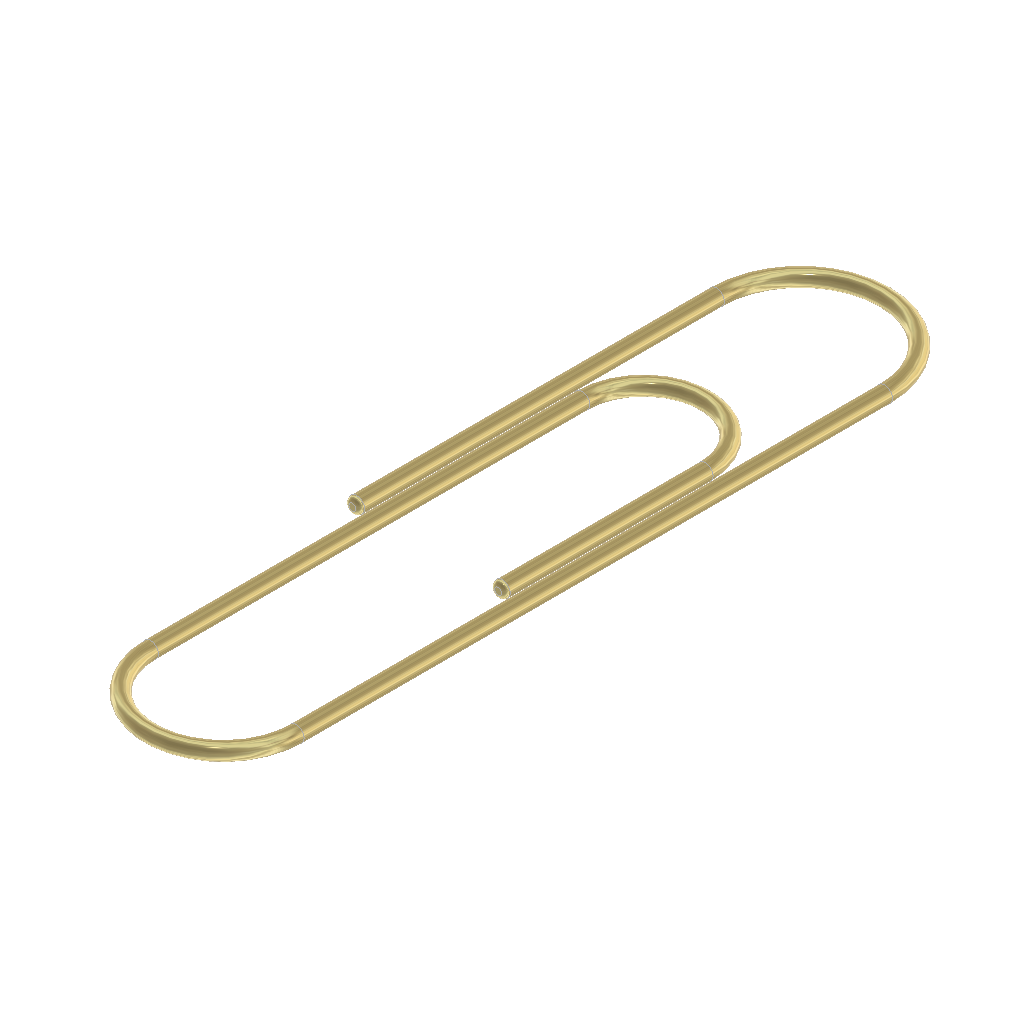
Paper Clip (Autodesk Fusion 360 design; units mm, degrees)
part number: 2026-09-26-18-15-15-186
Autodesk Fusion 360 part; units mm, degrees
sketch "path" plane through (0, 0, 0) normal (0, 0, 1) x (1, 0, 0)
  line L0 (0, 0) -> (0, 16.25)
  line L1 (7.5, 16.25) -> (7.5, -10)
  line L2 (1, -10) -> (1, 9.25)
  line L3 (6.5, 9.25) -> (6.5, 0)
  arc A0 (7.5, 16.25) -> (0, 16.25) centre (3.75, 16.25) ccw
  arc A1 (6.5, 9.25) -> (1, 9.25) centre (3.75, 9.25) ccw
  arc A2 (1, -10) -> (7.5, -10) centre (4.25, -10) ccw
  dimension "d1" = 16.25
  dimension "d2" = 7.5
  dimension "d3" = 26.25
  dimension "d4" = 6.5
  dimension "d5" = 19.25
  dimension "d6" = 5.5
  dimension "d7" = 9.25
  constraint coincident L0.start origin
  constraint vertical L0
  constraint tangent L0 A0
  constraint tangent L1 A0
  constraint tangent L2 A1
  constraint tangent L3 A1
  constraint tangent L1 A2
  constraint tangent L2 A2
  measures "d1" distance of L0.start L0.end
  measures "d2" distance of L0.end L1.start
  measures "d3" distance of L1.start L1.end
  measures "d4" distance of L1.end L2.start
  measures "d5" distance of L2.start L2.end
  measures "d6" distance of L2.end L3.start
  measures "d7" distance of L3.start L3.end
sketch "Profile" plane through (0, 0, 0) normal (0, 1, 0) x (1, 0, 0)
  circle A0 centre (0, 0) radius 0.35
  dimension "d8" = 0.7
  constraint coincident A0.centre origin
  measures "d8" diameter of A0
sweep "Sweep1" add profiles "Profile" path "path" along L0 A0 L1 A2 L2 A1 L3 section 1
fillet "Fillet1" radius 0.2 2 edges at (-0.3263, 0, 0.1266) (6.8263, 0, 0.1266)
